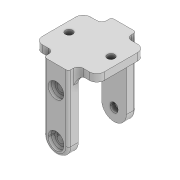
# Autodesk Inventor part: hobby motor mount
Saved by Autodesk Inventor 2022 (Build 260153000, 153)
## iProperties
Created: 2024-05-28
Part Number: hobby motor mount
Material: Generic
Document SubType Name: Modeling
Designer: david
Density: 1 g/cm^3
Appearance: Default
Author: david
Autodesk Inventor part; units mm, degrees
ref_plane "YZ Plane" through (0, 0, 0) normal (1, 0, 0) x (0, 1, 0)
ref_plane "XZ Plane" through (0, 0, 0) normal (0, 1, 0) x (-1, 0, 0)
ref_plane "XY Plane" through (0, 0, 0) normal (0, 0, 1) x (1, 0, 0)
sketch "Sketch1" plane through (0, 0, 0) normal (0, 1, 0) x (-1, 0, 0)
  line L0 (12.5, -9.75) -> (-12.5, -9.75)
  line L1 (-12.5, -9.75) -> (-12.5, 9.75)
  line L2 (-12.5, 9.75) -> (12.5, 9.75)
  line L3 (12.5, 9.75) -> (12.5, -9.75)
  line L4 (17.5, 0) -> (-17.5, 0) construction
  line L5 (0, -13.65) -> (0, 13.65) construction
  point P0 (0, 0)
  point P1 (0, 9.75)
  point P2 (-12.5, 0)
  dimension "d0" = 25
  dimension "d1" = 19.5
  constraints: 8 end point, 2 midpoint, 2 parallel, 1 horizontal, 1 horizontal alignment, 1 perpendicular, 1 vertical alignment
  measures "d0" distance of L1.end L2.end
  measures "d1" distance of L0.end L1.end
extrude "Extrusion1" add sketch "Sketch1" against normal blind 3
sketch "Sketch2" plane through (12.5, 0, -9.75) normal (0, 0, -1) x (-1, 0, 0)
  line L0 (12.5, 0) -> (12.5, -27) construction
  line L1 (17.5, 0) -> (17.5, -27)
  line L2 (7.5, -27) -> (7.5, 0)
  arc A0 (17.5, 0) -> (7.5, 0) centre (12.5, 0) ccw
  arc A1 (7.5, -27) -> (17.5, -27) centre (12.5, -27) ccw
  line L3 (0, 0) -> (25, 0) projected
  point P0 (12.5, -13.5)
  dimension "d4" = 27
  dimension "d5" = 10
  constraints: 8 end point, 4 point on circle, 4 tangent, 2 centre point, 1 midpoint, 1 parallel, 1 vertical
  measures "d4" distance of L0.start L0.end
  measures "d5" diameter of A1
extrude "Extrusion2" add sketch "Sketch2" along normal blind 4 contours L1 A1 L2 L3
sketch "Sketch3" plane through (12.5, 0, -13.75) normal (0, 0, -1) x (-1, 0, 0)
  line L0 (12.5, -27.25) -> (12.5, -26.75) construction
  line L1 (14.1, -27.25) -> (14.1, -26.75)
  line L2 (10.9, -26.75) -> (10.9, -27.25)
  arc A0 (10.9, -27.25) -> (14.1, -27.25) centre (12.5, -27.25) ccw
  arc A1 (14.1, -26.75) -> (10.9, -26.75) centre (12.5, -26.75) ccw
  arc A2 (7.5, -27) -> (17.5, -27) centre (12.5, -27) ccw projected
  point P0 (12.5, 0)
  dimension "d9" = 0.5
  dimension "d10" = 3.2
  constraints: 8 end point, 4 point on circle, 4 tangent, 2 centre point, 2 coincident, 1 midpoint, 1 parallel, 1 vertical
  measures "d9" distance of L0.start L0.end
  measures "d10" diameter of A0
extrude "Extrusion3" cut sketch "Sketch3" against normal through all
sketch "Sketch6" plane through (12.5, 0, -13.75) normal (0, 0, -1) x (-1, 0, 0)
  line L0 (14.1, -27.25) -> (14.1, -26.75) projected
  arc A0 (14.1, -26.75) -> (10.9, -26.75) centre (12.5, -26.75) ccw projected
  line L1 (10.9, -26.75) -> (10.9, -27.25) projected
  arc A1 (10.9, -27.25) -> (14.1, -27.25) centre (12.5, -27.25) ccw projected
  arc A2 (7.5, -27) -> (17.5, -27) centre (12.5, -27) ccw projected
  line L2 (7.5, -27) -> (7.5, 0) projected
  line L3 (7.5, 0) -> (17.5, 0) projected
  line L4 (17.5, 0) -> (17.5, -27) projected
  line L5 (9.35, -27.25) -> (9.35, -26.75)
  arc A3 (15.65, -26.75) -> (9.35, -26.75) centre (12.5, -26.75) ccw
  line L6 (15.65, -26.75) -> (15.65, -27.25)
  arc A4 (9.35, -27.25) -> (15.65, -27.25) centre (12.5, -27.25) ccw
  point P0 (12.5, 0)
  dimension "d33" = 6.3
  constraints: 4 end point, 4 point on circle, 2 centre point, 3 other
  measures "d33" distance from line of L6.start L5
extrude "Extrusion4" cut sketch "Sketch6" against normal blind 2 contours L5 A3 L6 A4
sketch "Sketch4" plane through (12.5, 0, -13.75) normal (0, 0, -1) x (-1, 0, 0)
  arc A0 (7.5, -27) -> (17.5, -27) centre (12.5, -27) ccw projected
  line L0 (7.5, -27) -> (7.5, 0) projected
  line L1 (7.5, 0) -> (17.5, 0) projected
  line L2 (17.5, 0) -> (17.5, -27) projected
  arc A1 (9.35, -27.25) -> (15.65, -27.25) centre (12.5, -27.25) ccw projected
  line L3 (15.65, -27.25) -> (15.65, -26.75) projected
  arc A2 (15.65, -26.75) -> (9.35, -26.75) centre (12.5, -26.75) ccw projected
  line L4 (9.35, -26.75) -> (9.35, -27.25) projected
  point P0 (12.5, 0)
  point P1 (12.5, -9.25)
  dimension "d37" = 18
  constraints: 1 vertical alignment
  measures "d37" distance of point (12.5, -9.25) A1.centre
hole "Hole1" at (0, -9.25, -13.75) direction (0, 0, 1) diameter 3.2 end through all counterbore diameter 6.3 counterbore depth 2
mirror "Mirror1" about plane through (0, 0, 0) normal (0, 0, 1) of "Extrusion2", "Hole1", "Extrusion3", "Extrusion4"
fillet "Fillet1" radius 3 4 edges at (-12.5, -1.5, 9.75) (-12.5, -1.5, -9.75) (12.5, -1.5, -9.75) (12.5, -1.5, 9.75)
fillet "Fillet2" radius 2 4 edges at (-5, -1.5, -9.75) (-5, -1.5, 9.75) (5, -1.5, 9.75) (5, -1.5, -9.75)
fillet "Fillet3" radius 1 6 edges at (0, -32, 13.75) (5, -13.5, 13.75) (-5, -13.5, 13.75) (0, -32, -13.75) (5, -13.5, -13.75) (-5, -13.5, -13.75)
fillet "Fillet4" radius 3 6 edges at (0, -3, -9.75) (-5, -3, -10.75) (5, -3, -10.75) (0, -3, 9.75) (-5, -3, 10.75) (5, -3, 10.75)
sketch "Sketch5" plane through (0, -3, 0) normal (0, -1, 0) x (1, 0, 0)
  line L0 (-8.5, 0) -> (8.5, 0)
  line L1 (-12.5, 6.75) -> (-12.5, -6.75) projected
  point P0 (0, 0)
  point P1 (0, 0)
  dimension "d25" = 4
  constraints: 3 coincident, 2 end point, 1 horizontal, 1 midpoint
  measures "d25" distance from line of L1 L0.start
hole "Hole2" at (-8.5, -3, 0) at (8.5, -3, 0) direction (0, 1, 0) diameter 3 depth 5 tip angle 118
fillet "Fillet5" radius 0.7 10 edges at (0, -12.4, 11.75) (-3.15, -27, 11.75) (0, -30.4, 11.75) (3.15, -27, 11.75) (0, -23.6, 11.75) (3.15, -27, -11.75) (0, -23.6, -11.75) (-3.15, -27, -11.75) (0, -30.4, -11.75) (0, -12.4, -11.75)
body "Solid1"
